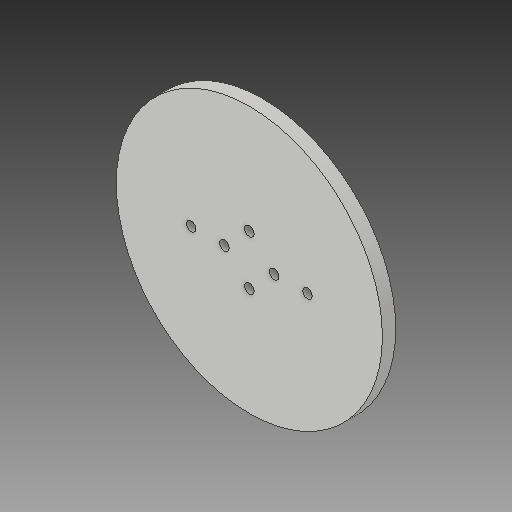
# Autodesk Inventor part: thrusterMount
Saved by Autodesk Inventor 2018 (Build 220112000, 112)
## iProperties
Created: 2020-01-10
Part Number: thrusterMount
Material: Generic
Document SubType Name: Modeling
Designer: anirudh
Density: 1 g/cm^3
Appearance: Default
Author: anirudh
Autodesk Inventor part; units mm, degrees
ref_plane "YZ Plane" through (0, 0, 0) normal (1, 0, 0) x (0, 1, 0)
ref_plane "XZ Plane" through (0, 0, 0) normal (0, 1, 0) x (-1, 0, 0)
ref_plane "XY Plane" through (0, 0, 0) normal (0, 0, 1) x (1, 0, 0)
sketch "Sketch1" plane through (0, 0, 0) normal (0, 0, 1) x (1, 0, 0)
  circle A0 centre (0, 0) radius 38.1
  circle A1 centre (0, -9.5) radius 1.85
  circle A2 centre (9.5, 0) radius 1.85
  circle A3 centre (0, 9.5) radius 1.85
  circle A4 centre (-9.5, 0) radius 1.85
  circle A5 centre (-22.1996, 0) radius 1.8
  circle A6 centre (-22.1996, 0) radius 1.8
  circle A7 centre (22.1996, 0) radius 1.8
  circle A8 centre (22.1996, 0) radius 1.8
  point P0 (-6.7175, 6.7175)
  point P1 (6.7175, -6.7175)
  point P2 (6.7175, 6.7175)
  constraints: 9 centre point, 3 coincident
extrude "Extrusion1" add sketch "Sketch1" along normal blind 5.08
sketch "Sketch2" plane through (0, 0, 5.08) normal (0, 0, 1) x (1, 0, 0)
  circle A0 centre (0, 0) radius 38.1
  circle A1 centre (0, 0) radius 50.8
  dimension "d3" = 101.6
  constraints: 2 centre point, 2 coincident
  measures "d3" diameter of A1
extrude "Extrusion2" add sketch "Sketch2" against normal blind 5.08
sketch "Sketch4" plane through (0, 0, 5.08) normal (0, 0, 1) x (1, 0, 0)
  circle A0 centre (-9.5, 0) radius 1.85 projected
  circle A1 centre (-9.5, 0) radius 1.8
  circle A2 centre (0, 9.5) radius 1.85 projected
  circle A3 centre (0, 9.5) radius 1.8
  circle A4 centre (0, -9.5) radius 1.85 projected
  circle A5 centre (0, -9.5) radius 1.8
  circle A6 centre (9.5, 0) radius 1.85 projected
  circle A7 centre (9.5, 0) radius 1.8
  point P0 (0, 0)
  dimension "d6" = 3.6
  dimension "d7" = 3.6
  dimension "d8" = 3.6
  dimension "d9" = 3.6
  constraints: 4 centre point, 4 coincident
  measures "d6" diameter of A1
  measures "d7" diameter of A3
  measures "d8" diameter of A5
  measures "d9" diameter of A7
body "Solid1"
